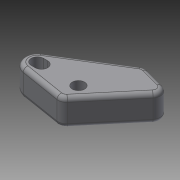
# Autodesk Inventor part: brake
Saved by Autodesk Inventor 2018 (Build 220112000, 112)
## iProperties
Created: 2019-02-20
Part Number: brake
Material: 一般
Document SubType Name: Modeling
Designer: ku_sk
Density: 1 g/cm^3
Appearance: 既定
Author: ku_sk
Autodesk Inventor part; units mm, degrees
ref_plane "YZ Plane" through (0, 0, 0) normal (1, 0, 0) x (0, 1, 0)
ref_plane "XZ Plane" through (0, 0, 0) normal (0, 1, 0) x (-1, 0, 0)
ref_plane "XY Plane" through (0, 0, 0) normal (0, 0, 1) x (1, 0, 0)
sketch "スケッチ1" plane through (0, 0, 0) normal (0, 0, 1) x (1, 0, 0)
  arc A0 (-1.5776, 2.5517) -> (-0.4828, -2.9609) centre (0, 0) ccw
  line L0 (-1.5776, 2.5517) -> (13.2904, 11.7436)
  line L1 (20.7039, 7.4628) -> (11.1913, -3.8738)
  line L2 (9.3374, -4.5621) -> (-0.4828, -2.9609)
  arc A1 (20.7039, 7.4628) -> (19.6894, 10.6802) centre (19.1718, 8.7484) ccw
  arc A2 (9.3374, -4.5621) -> (11.1913, -3.8738) centre (9.6593, -2.5882) ccw
  line L3 (0, 0) -> (9.6593, -2.5882)
  line L4 (9.6593, -2.5882) -> (19.1718, 8.7484)
  line L5 (-8.5052, 0) -> (26.6017, 0) projected
  line L6 (19.6894, 10.6802) -> (14.8598, 11.9743)
  arc A3 (14.8598, 11.9743) -> (13.2904, 11.7436) centre (14.3421, 10.0425) ccw
  line L7 (19.1718, 8.7484) -> (14.3421, 10.0425)
  line L8 (14.3421, 10.0425) -> (0, 0)
  dimension "d0" = 2
  dimension "d18" = 15
  dimension "d19" = 115
  dimension "d20" = 3
  dimension "d21" = 2
  dimension "d22" = 130
  dimension "d23" = 65
  dimension "d24" = 10
  dimension "d25" = 5
  constraints: 16 end point, 8 point on circle, 8 tangent, 4 centre point, 1 coincident, 1 equal radius
  measures "d0" radius of A1
  measures "d18" angle of L5 L3
  measures "d19" angle of L3 L4
  measures "d20" radius of A0
  measures "d21" radius of A3
  measures "d22" angle of L8 L7
  measures "d23" angle of L7 L4
  measures "d24" distance of L3.start L3.end
  measures "d25" distance of L4.end L7.end
extrude "押し出し1" add sketch "スケッチ1" along normal blind 6.5
sketch "スケッチ3" plane through (0, 0, 6.5) normal (0, 0, 1) x (1, 0, 0)
  line L0 (0, 0) -> (1, 0) construction
  line L1 (0, 1.5) -> (1, 1.5)
  line L2 (1, -1.5) -> (0, -1.5)
  arc A0 (0, 1.5) -> (0, -1.5) centre (0, 0) ccw
  arc A1 (1, -1.5) -> (1, 1.5) centre (1, 0) ccw
  point P0 (0.5, 0)
  dimension "d7" = 3
  dimension "d8" = 1
  constraints: 8 end point, 4 point on circle, 4 tangent, 2 centre point, 1 horizontal, 1 midpoint, 1 parallel
  measures "d7" distance between parallel lines of L1 L2
  measures "d8" distance of L0.start L0.end
extrude "押し出し3" cut sketch "スケッチ3" against normal through all
sketch "スケッチ5" plane through (0, 0, 6.5) normal (0, 0, 1) x (1, 0, 0)
  circle A0 centre (10, 0) radius 1.5
  line L0 (-7.8344, 0) -> (26.0061, 0) projected
  point P0 (0, 0)
  dimension "d14" = 3
  dimension "d15" = 10
  constraints: 1 centre point, 1 point on line
  measures "d14" diameter of A0
  measures "d15" distance of point (0, 0) A0.centre
extrude "押し出し5" cut sketch "スケッチ5" against normal through all
fillet "フィレット2" radius 1 16 edges at (-2.9425, -0.5844, 6.5) (4.4273, -3.7615, 6.5) (10.3554, -4.4631, 6.5) (15.9476, 1.7945, 6.5) (21.0792, 9.3498, 6.5) (17.2746, 11.3273, 6.5) (14.0513, 12.0212, 6.5) (5.8564, 7.1477, 6.5) (-2.9425, -0.5844, 0) (4.4273, -3.7615, 0) (10.3554, -4.4631, 0) (15.9476, 1.7945, 0) (21.0792, 9.3498, 0) (17.2746, 11.3273, 0) (14.0513, 12.0212, 0) (5.8564, 7.1477, 0)
